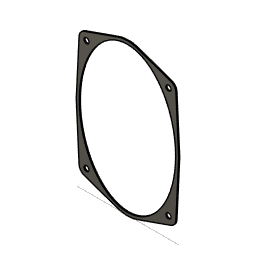
Speaker Template (Autodesk Fusion 360 design; units mm, degrees)
Autodesk Fusion 360 part; units mm, degrees
sketch "Sketch1" plane through (0, 0, 0) normal (0, 0, 1) x (1, 0, 0)
  line L0 (-50, 74) -> (50, 74) construction
  line L1 (50, 74) -> (50, -74) construction
  line L2 (50, -74) -> (-50, -74) construction
  line L3 (-50, -74) -> (-50, 74) construction
  line L4 (-50, 74) -> (50, -74) construction
  line L5 (50, 74) -> (-50, -74) construction
  circle A0 centre (-40, 54) radius 2.5
  circle A1 centre (40, 54) radius 2.5
  circle A2 centre (-40, -54) radius 2.5
  circle A3 centre (40, -54) radius 2.5
  line L6 (0, 74) -> (0, 0)
  line L7 (-50, 0) -> (0, 0)
  line L8 (50, 0) -> (47.2407, 54.3675)
  arc A4 (9.5249, 72.3996) -> (0, 74) centre (0, 44.8559) ccw
  line L9 (9.5249, 72.3996) -> (42.4047, 60.8396)
  arc A5 (47.2407, 54.3675) -> (42.4047, 60.8396) centre (40, 54) ccw
  arc A6 (0, -74) -> (9.5249, -72.3996) centre (0, -44.8559) ccw
  line L10 (9.5249, -72.3996) -> (42.4047, -60.8396)
  arc A7 (42.4047, -60.8396) -> (47.2407, -54.3675) centre (40, -54) ccw
  line L11 (50, 0) -> (47.2407, -54.3675)
  arc A8 (-9.5249, -72.3996) -> (0, -74) centre (0, -44.8559) ccw
  line L12 (-9.5249, -72.3996) -> (-42.4047, -60.8396)
  arc A9 (-47.2407, -54.3675) -> (-42.4047, -60.8396) centre (-40, -54) ccw
  line L13 (-50, 0) -> (-47.2407, -54.3675)
  line L14 (-50, 0) -> (-47.2407, 54.3675)
  arc A10 (0, 74) -> (-9.5249, 72.3996) centre (0, 44.8559) ccw
  line L15 (-9.5249, 72.3996) -> (-42.4047, 60.8396)
  arc A11 (-42.4047, 60.8396) -> (-47.2407, 54.3675) centre (-40, 54) ccw
  dimension "d1" = 100
  dimension "d2" = 148
  dimension "d3" = 5
  dimension "d4" = 54
  dimension "d5" = 40
  dimension "d8" = 80
  dimension "d9" = -108
  dimension "d10" = 14.5
  constraint horizontal L0
  constraint perpendicular L0 L1
  constraint parallel L0 L2
  constraint parallel L1 L3
  constraint coincident L4 L6.end
  constraint coincident L5 L6.end
  constraint coincident L6.end L7.end
  constraint midpoint L0 L6.start
  constraint midpoint L3 L7.start
  constraint concentric A1 A5
  constraint midpoint L1 L8.start
  constraint tangent L8 A5
  constraint coincident L6 A4.centre
  constraint tangent L0 A4
  constraint tangent L9 A5
  constraint symmetric L6.start L7 A6.start
  constraint symmetric L7 L8.start L11.start
  constraint symmetric L7 L8.end A7.end
  constraint symmetric L7 A4.start A6.end
  constraint symmetric L7 A4 A6
  constraint symmetric L7 L9.end L10.end
  constraint symmetric L7 A5 A7
  constraint symmetric A4.end L6 A10.start
  constraint symmetric L6 L8.start L7.start
  constraint symmetric L6 L8.end L14.end
  constraint symmetric L6 A4.start A10.end
  constraint symmetric L6 A4 A10
  constraint symmetric L6 L9.end L15.end
  constraint symmetric L6 A5 A11
  constraint symmetric L6 A6.end A8.start
  constraint symmetric L6 A6.start A8.end
  constraint symmetric L6 A6 A8
  constraint symmetric L6 L10.end L12.end
  constraint symmetric L6 A7.end A9.start
  constraint symmetric L6 A7 A9
  measures "d1" distance of L1.end L2.end
  measures "d2" distance of L0.end L1.end
  measures "d3" diameter of A0
  measures "d4" vertical distance of L6.end A0.centre
  measures "d5" horizontal distance of L6.end A0.centre
  measures "d10" diameter of A5
sketch "Sketch2" plane through (0, 0, 0) normal (0, 0, 1) x (1, 0, 0)
  ellipse E0 centre (0, 0) end of major axis (0, 71) minor radius 47
  line L0 (0, -71) -> (0, 71)
  line L1 (47, 0) -> (-47, 0)
  dimension "d11" = 142
  dimension "d12" = 94
  constraint coincident E0 L0.start
  constraint coincident E0 L0.end
  constraint coincident E0 L1.start
  constraint coincident E0 L1.end
  constraint coincident E0.centre origin
  constraint vertical L0
  measures "d11" distance of E0
extrude "Extrude1" add sketch "Sketch1" along normal blind 1
extrude "Extrude2" cut sketch "Sketch2" along normal through all
equation "d4 = ( 108 / 2 ) * 1 mm"
